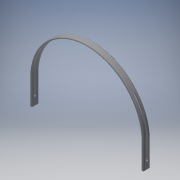
# Autodesk Inventor part: kinect_ring_fixt
Saved by Autodesk Inventor 2019 (Build 230136000, 136)
## iProperties
Created: 2024-05-02
Part Number: kinect_ring_fixt
Material: Generisch
Document SubType Name: Modeling
Designer: nic
Density: 1 g/cm^3
Appearance: Vorgabe
Author: nic
Autodesk Inventor part; units mm, degrees
ref_plane "YZ Plane" through (0, 0, 0) normal (1, 0, 0) x (0, 1, 0)
ref_plane "XZ Plane" through (0, 0, 0) normal (0, 1, 0) x (-1, 0, 0)
ref_plane "XY Plane" through (0, 0, 0) normal (0, 0, 1) x (1, 0, 0)
sketch "Skizze1" plane through (0, 0, 0) normal (0, 0, 1) x (1, 0, 0)
  spline S0 degree 3 poles (-105.8822, 140.749) (-105.8788, 141.4909) (-105.8763, 142.2326) (-105.8735, 144.075) (-105.8756, 145.1221) (-105.8847, 146.6639) (-105.8907, 147.2231) (-105.9017, 147.9704) (-105.9068, 148.1673) (-105.9095, 148.1777) knots -2.336079 -2.336079 -2.336079 -2.336079 -2.113673 -2.113673 -1.757823 -1.757823 -1.463963 -1.463963 -1.177437 -1.177437 -1.177437 -1.177437 construction
  spline S1 degree 3 poles (104.5344, 148.1777) (104.5332, 148.173) (104.5315, 148.1305) (104.5239, 147.8283) (104.5158, 147.3114) (104.5046, 145.9435) (104.5009, 145.1718) (104.499, 143.6365) (104.4997, 142.9127) (104.5031, 141.6997) (104.5049, 141.2244) (104.5071, 140.749) knots -1.158642 -1.158642 -1.158642 -1.158642 -1.029023 -1.029023 -0.666944 -0.666944 -0.370525 -0.370525 -0.142509 -0.142509 0 0 0 0 construction
  arc A0 (104.5071, 140.749) -> (-105.8822, 139.0208) centre (-0.6196, 131.612) ccw
  line L0 (104.5071, 140.749) -> (104.5071, 82.9614)
  line L1 (-105.8822, 82.9614) -> (-105.8822, 139.0208)
  arc A1 (109.3627, 139.0208) -> (-110.305, 139.0208) centre (-0.4712, 129.2808) ccw
  line L2 (109.3627, 139.0208) -> (109.3627, 82.9614)
  line L3 (-110.305, 82.9614) -> (-110.305, 139.0208)
  line L4 (109.3627, 82.9614) -> (104.5071, 82.9614)
  line L5 (-105.8822, 82.9614) -> (-110.305, 82.9614)
  point P0 (0, 0)
  constraints: 12 end point, 4 point on circle, 2 centre point, 2 parallel
extrude "Extrusion1" add sketch "Skizze1" along normal blind 12
sketch "Skizze2" plane through (-110.305, 82.9614, 0) normal (-1, 0, 0) x (0, 0, 1)
  line L0 (0, 0) -> (0, 56.0595) construction
  line L1 (0, 0) -> (12, 0) construction
  line L2 (12, 56.0595) -> (12, 0) construction
  line L3 (0, 56.0595) -> (12, 56.0595) construction
  line L4 (12, 56.0595) -> (12, 156.5843) construction
  line L5 (0, 56.0595) -> (0, 56.0595) construction
  line L6 (0, 56.0595) -> (12, 56.0595) construction
  line L7 (12, 56.0595) -> (12, 56.0595) construction
  line L8 (0, 56.0595) -> (12, 56.0595) construction
  line L9 (6, 14.5203) -> (6, 94.7602) construction
  line L10 (7.75, 16.2703) -> (7.75, 93.0102)
  line L11 (4.25, 93.0102) -> (4.25, 16.2703)
  arc A0 (4.25, 16.2703) -> (7.75, 16.2703) centre (6, 16.2703) ccw
  line L12 (6, 54.6403) -> (6, 115.372) construction
  line L13 (7.75, 56.3903) -> (7.75, 113.622)
  line L14 (4.25, 113.622) -> (4.25, 56.3903)
  arc A1 (7.75, 113.622) -> (4.25, 113.622) centre (6, 113.622) ccw
  arc A2 (4.25, 56.3903) -> (4.2816, 56.0595) centre (6, 56.3903) ccw
  arc A3 (7.7184, 56.0595) -> (7.75, 56.3903) centre (6, 56.3903) ccw
  line L15 (6, 16.2703) -> (6, 113.622) construction
  line L16 (7.75, 16.2703) -> (7.75, 113.622)
  line L17 (4.25, 113.622) -> (4.25, 16.2703)
  arc A4 (4.25, 16.2703) -> (7.75, 16.2703) centre (6, 16.2703) ccw
  arc A5 (7.75, 113.622) -> (4.25, 113.622) centre (6, 113.622) ccw
  point P0 (6, 85.0062)
  point P1 (6, 64.9462)
  constraints: 24 end point, 14 point on circle, 10 tangent, 7 point on line, 6 centre point, 3 midpoint, 3 parallel, 1 collinear, 1 concentric, 1 vertical
extrude "Extrusion3" cut sketch "Skizze2" against normal through all
fillet "Rundung1" radius 2 8 edges at (-0.4712, 239.5457, 0) (-0.4712, 239.5457, 12) (-110.305, 110.9911, 12) (-110.305, 110.9911, 0) (-110.305, 82.9614, 6) (109.3627, 110.9911, 12) (109.3627, 110.9911, 0) (109.3627, 82.9614, 6)
